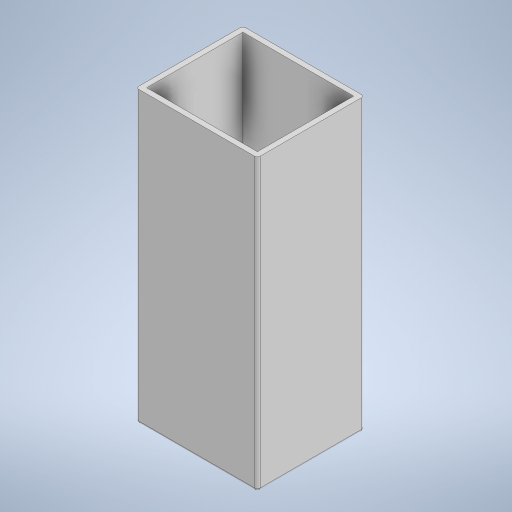
# Autodesk Inventor part: Battery Box Top
Saved by Autodesk Inventor 2024 (Build 280153000, 153)
## iProperties
Created: 2023-07-25
Part Number: Battery Box Top
Material: Generic
Document SubType Name: Modeling
Designer: techn
Density: 1 g/cm^3
Appearance: Default
Author: techn
## iProperties of the stored document Battery Box Top_3DPrint.ipt
Created: 2023-07-25
Part Number: Battery Box Top_3DPrint
Material: Generic
Document SubType Name: Modeling
Designer: techn
Density: 1 g/cm^3
Appearance: Default
Author: techn
Autodesk Inventor part; units mm, degrees
ref_plane "YZ Plane" through (0, 0, 0) normal (1, 0, 0) x (0, 1, 0)
ref_plane "XZ Plane" through (0, 0, 0) normal (0, 1, 0) x (-1, 0, 0)
ref_plane "XY Plane" through (0, 0, 0) normal (0, 0, 1) x (1, 0, 0)
sketch "Sketch1" plane through (0, 0, 0) normal (0, 1, 0) x (-1, 0, 0)
  point P0 (0, 0)
sketch "Sketch2" plane through (0, 0, 0) normal (0, 1, 0) x (-1, 0, 0)
  line L0 (5.8709, 8.8623) -> (-86.1291, 8.8623)
  line L1 (-86.1291, 8.8623) -> (-86.1291, 89.8623)
  line L2 (-86.1291, 89.8623) -> (5.8709, 89.8623)
  line L3 (5.8709, 89.8623) -> (5.8709, 8.8623)
  line L4 (1.8709, 85.8623) -> (-82.1291, 85.8623)
  line L5 (-82.1291, 85.8623) -> (-82.1291, 12.8623)
  line L6 (-82.1291, 12.8623) -> (1.8709, 12.8623)
  line L7 (1.8709, 12.8623) -> (1.8709, 85.8623)
  point P0 (0, 0)
  dimension "d0" = 92
  dimension "d1" = 81
  dimension "d4" = 84
  dimension "d5" = 73
  constraints: 16 end point, 4 parallel, 2 horizontal, 2 perpendicular
  measures "d0" distance of L1.end L2.end
  measures "d1" distance of L0.end L1.end
  measures "d4" distance of L6.end L5.end
  measures "d5" distance of L5.end L4.end
extrude "Extrusion1" add sketch "Sketch2" along normal blind 4 contours L0 L1 L2 L3 | L7 L6 L5 L4
sketch "Sketch3" plane through (0, 4, 0) normal (0, 1, 0) x (1, 0, 0)
  line L0 (-5.8709, -89.8623) -> (86.1291, -89.8623) projected
  line L1 (-1.8709, -89.8623) -> (2.1291, -89.8623) construction
  line L2 (-1.8709, -85.8623) -> (82.1291, -85.8623)
  line L3 (82.1291, -85.8623) -> (82.1291, -12.8623)
  line L4 (82.1291, -12.8623) -> (-1.8709, -12.8623)
  line L5 (-1.8709, -12.8623) -> (-1.8709, -85.8623)
  line L6 (86.1291, -89.8623) -> (86.1291, -8.8623) projected
  line L7 (-5.8709, -89.8623) -> (86.1291, -89.8623)
  line L8 (86.1291, -89.8623) -> (86.1291, -8.8623)
  line L9 (86.1291, -8.8623) -> (-5.8709, -8.8623)
  line L10 (-5.8709, -8.8623) -> (-5.8709, -89.8623)
  point P0 (0, 0)
  dimension "d9" = 4
  dimension "d11" = 84
  dimension "d12" = 73
  constraints: 18 end point, 4 parallel, 3 horizontal, 2 perpendicular, 1 point on line
  measures "d9" distance of L1.start L2.start
  measures "d11" distance of L4.end L3.end
  measures "d12" distance of L3.end L2.end
extrude "Extrusion2" add sketch "Sketch3" along normal blind 216
fillet "Fillet1" radius 2 8 edges at (86.1291, 110, 89.8623) (86.1291, 110, 8.8623) (-5.8709, 110, 8.8623) (-5.8709, 110, 89.8623) (40.1291, 0, 89.8623) (86.1291, 0, 49.3623) (40.1291, 0, 8.8623) (-5.8709, 0, 49.3623)
body "Solid1"
